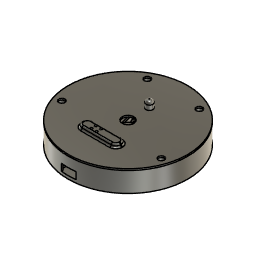
ViveTrackerPogoBatteryV2 (Autodesk Fusion 360 design; units mm, degrees)
Autodesk Fusion 360 part; units mm, degrees
sketch "CaseBase" plane through (0, 0, 0) normal (0, 0, 1) x (1, 0, 0)
  circle A0 centre (0, 0) radius 39
  dimension "d3" = 78
  constraint coincident A0.centre origin
  measures "d3" diameter of A0
sketch "Charging Module" plane through (0, 0, 0) normal (0, 0, 1) x (1, 0, 0)
  line L0 (-10, 37.25, 1) -> (10, 37.25, 1)
  line L1 (10, 37.25, 1) -> (10, 12.25, 1)
  line L2 (10, 12.25, 1) -> (-10, 12.25, 1)
  line L3 (-10, 12.25, 1) -> (-10, 37.25, 1)
  dimension "d9" = 25
  dimension "d10" = 20
sketch "Batteries" plane through (0, 0, 0) normal (0, 0, 1) x (1, 0, 0)
  line L0 (0, 2.5) -> (0, 20)
  line L1 (14.1047, 22.1855, 1) -> (1.1638, -26.1107, 1)
  line L2 (20.4823, -31.2871, 1) -> (33.4233, 17.0092, 1)
  line L3 (33.4233, 17.0092, 1) -> (14.1047, 22.1855, 1)
  line L4 (1.1638, -26.1107, 1) -> (20.4823, -31.2871, 1)
  line L5 (-1.1638, -26.1107, 1) -> (-20.4823, -31.2871, 1)
  line L6 (-20.4823, -31.2871, 1) -> (-33.4233, 17.0092, 1)
  line L7 (-14.1047, 22.1855, 1) -> (-1.1638, -26.1107, 1)
  line L8 (-33.4233, 17.0092, 1) -> (-14.1047, 22.1855, 1)
  dimension "d52" = 20
  dimension "d53" = 50
extrude "Extrude6" add sketch "Charging Module" along normal blind 2 contours L0 L1 L2 L3 in plane through (0, 0, 1) normal (0, 0, 1) makes body 1
sketch "Sketch11" plane through (0, 0, 3) normal (0, 0, 1) x (-1, 0, 0)
  line L0 (10, -12.25) -> (-10, -12.25)
  line L1 (-10, -12.25) -> (-10, -37.25)
  line L2 (-10, -37.25) -> (10, -37.25)
  line L3 (10, -37.25) -> (10, -12.25)
  line L4 (4.508, -37.25) -> (-4.492, -37.25)
  line L5 (-4.492, -37.25) -> (-4.492, -29.85)
  line L6 (-4.492, -29.85) -> (4.508, -29.85)
  line L7 (4.508, -29.85) -> (4.508, -37.25)
  dimension "d64" = 9
  dimension "d65" = 7.4
  constraint coincident L2 L4.start
  measures "d64" distance of L4.start L4.end
  measures "d65" distance of L4.start L6.end
extrude "Extrude12" add sketch "Sketch11" along normal blind 3 contours L2 L4 L5 L6 L7 bodies 1
extrude "Extrude7" add sketch "CaseBase" along normal blind 13 separate body makes body 2
shell "Shell2" thickness 1 removed faces 1 at (-7.0083, -19.4245, 13) on bodies 2
sketch "ScrewHoleThing" plane through (0, 0, 0) normal (0, 0, 1) x (1, 0, 0)
  circle A0 centre (0, 0) radius 6
  dimension "d28" = 12
  constraint coincident A0.centre origin
  measures "d28" diameter of A0
extrude "Extrude8" add sketch "ScrewHoleThing" along normal blind 8.5 bodies 2
hole "Hole5" at (0, 0, 8.5) direction (0, 0, -1) diameter 7.25 depth 10 tip angle 180 bodies 2
sketch "OG Comparison" plane through (0, 0, 0) normal (0, 0, 1) x (1, 0, 0)
  circle A0 centre (0, 0) radius 45
  dimension "d51" = 90
  constraint coincident A0.centre origin
  measures "d51" diameter of A0
extrude "Extrude9" add sketch "Batteries" along normal blind 10 separate body contours L1 L2 L3 L4 | L5 L6 L7 L8 in plane through (0, 0, 1) normal (0, 0, 1) makes body 3 at (16.2306, 4.3613, 1) makes body 4 at (-18.3565, -13.4629, 1)
sketch "SwitchCutout" plane through (0, 0, 0) normal (0, 1, 0) x (1, 0, 0)
  line L0 (-4.75, -6.5, -40.0305) -> (4.75, -6.5, -40.0305)
  line L1 (4.75, -6.5, -40.0305) -> (4.75, -2, -40.0305)
  line L2 (4.75, -2, -40.0305) -> (-4.75, -2, -40.0305)
  line L3 (-4.75, -2, -40.0305) -> (-4.75, -6.5, -40.0305)
  dimension "d56" = 9.5
  dimension "d57" = 4.5
extrude "Extrude10" cut sketch "SwitchCutout" along normal blind 4 contours L0 L1 L2 L3 in plane through (0, -40.0305, 0) normal (0, 1, 0) bodies 4 3 2
sketch "Sketch10" plane through (0, 0, 1) normal (0, 0, 1) x (-1, 0, 0)
  line L0 (-6, 38.15) -> (6, 38.15)
  line L1 (6, 38.15) -> (6, 32.15)
  line L2 (6, 32.15) -> (-6, 32.15)
  line L3 (-6, 32.15) -> (-6, 38.15)
  circle A0 centre (0, 0) radius 6
  circle A1 centre (0, 0) radius 38
  dimension "d60" = 12
  dimension "d61" = 6
  constraint horizontal L0
  constraint vertical L1
  constraint horizontal L2
  constraint vertical L3
  measures "d60" distance of L0.start L0.end
  measures "d61" distance of L0.start L2.end
extrude "Extrude11" add sketch "Sketch10" along normal blind 1 contours L1 L2 L3 A1 picked at (0.6692, 34.0823) bodies 2
sketch "Sketch12" plane through (0, 0, 1) normal (0, 0, 1) x (-1, 0, 0)
  line L0 (6, 37.5233) -> (6, 32.15)
  line L1 (6, 32.15) -> (-6, 32.15)
  line L2 (-6, 32.15) -> (-6, 37.5233)
  arc A0 (-6, 37.5233) -> (6, 37.5233) centre (0, 0) ccw
  line L3 (13.9813, -22.3263) -> (13.0154, -22.5851)
  line L4 (13.0154, -22.5851) -> (0.0745, 25.7112)
  line L5 (0.0745, 25.7112) -> (1.0404, 25.97)
  line L6 (1.0404, 25.97) -> (13.9813, -22.3263)
  line L7 (22.2661, 31.9239) -> (35.2071, -16.3724)
  line L8 (35.2071, -16.3724) -> (34.2411, -16.6313)
  line L9 (21.3002, 31.665) -> (22.2661, 31.9239)
  line L10 (34.2411, -16.6313) -> (21.3002, 31.665)
  circle A1 centre (0, 0) radius 6
  line L11 (20.3106, 32.0212) -> (0.9921, 26.8448)
  line L12 (0.9921, 26.8448) -> (0.7333, 27.8107)
  line L13 (0.7333, 27.8107) -> (20.0518, 32.9871)
  line L14 (20.0518, 32.9871) -> (20.3106, 32.0212)
  line L15 (0, -2.5) -> (0, -20)
  line L16 (-20.3106, 32.0212) -> (-0.9921, 26.8448)
  line L17 (-0.9921, 26.8448) -> (-0.7333, 27.8107)
  line L18 (-20.0518, 32.9871) -> (-20.3106, 32.0212)
  line L19 (-0.7333, 27.8107) -> (-20.0518, 32.9871)
  line L20 (-34.2411, -16.6313) -> (-21.3002, 31.665)
  line L21 (-21.3002, 31.665) -> (-22.2661, 31.9239)
  line L22 (-35.2071, -16.3724) -> (-34.2411, -16.6313)
  line L23 (-22.2661, 31.9239) -> (-35.2071, -16.3724)
  line L24 (-1.0404, 25.97) -> (-13.9813, -22.3263)
  line L25 (-13.9813, -22.3263) -> (-13.0154, -22.5851)
  line L26 (-0.0745, 25.7112) -> (-1.0404, 25.97)
  line L27 (-13.0154, -22.5851) -> (-0.0745, 25.7112)
  dimension "d68" = 50
  dimension "d69" = 1
  dimension "d70" = 50
  dimension "d71" = 1
  dimension "d86" = 20
  dimension "d87" = 1
  constraint symmetric L3.start L15 L24.end
  constraint symmetric L3.end L15 L25.end
  constraint symmetric L4.end L15 L26.start
  constraint symmetric L5.end L15 L24.start
  constraint symmetric L8.end L15 L20.start
  constraint symmetric L7.start L15 L21.end
  constraint symmetric L7.end L15 L22.start
  constraint symmetric L9.start L15 L20.end
  constraint symmetric L11.start L15 L16.start
  constraint symmetric L11.end L15 L16.end
  constraint symmetric L12.end L15 L17.end
  constraint symmetric L13.end L15 L18.start
  measures "d68" distance of L3.start L5.end
  measures "d69" distance of L3.start L3.end
  measures "d70" distance of L7.start L7.end
  measures "d71" distance of L8.end L7.end
  measures "d86" distance of L11.start L11.end
  measures "d87" distance of L11.end L12.end
extrude "Extrude16" add sketch "Sketch12" along normal blind 4 contours A0 L11 L12 L13 L14 | A0 L7 L10 | A0 L16 L17 L18 L19 | A0 L20 L23 | L3 L4 L5 L6 | L24 L25 L26 L27 bodies 2
sketch "Sketch14" plane through (0, 0, 1) normal (0, 0, 1) x (-1, 0, 0)
  line L0 (10.7, -36.7464) -> (10.2816, -36.7464)
  line L1 (10.2816, -36.7464) -> (10.2816, -12.3822)
  line L2 (10.2816, -12.3822) -> (10.7, -12.3822)
  line L3 (10.7, -12.3822) -> (10.7, -36.7464)
  line L4 (13.0154, -22.5851) -> (0.0745, 25.7112)
  line L5 (-10.3, -12.3822) -> (-10.3, -36.7464)
  line L6 (-10.3, -36.7464) -> (-10.7184, -36.7464)
  line L7 (-10.7184, -12.3822) -> (-10.3, -12.3822)
  line L8 (-10.7184, -36.7464) -> (-10.7184, -12.3822)
  circle A0 centre (8.7853, -10.6413) radius 1
  circle A1 centre (-8.7147, -10.6413) radius 1
  dimension "d78" = 2
  dimension "d79" = 2
  constraint horizontal L0
  constraint vertical L1
  constraint horizontal L2
  constraint vertical L3
  constraint coincident L1.end L4
  constraint horizontal L6
  constraint vertical L8
  constraint horizontal L7
  constraint vertical L5
  measures "d78" diameter of A0
  measures "d79" diameter of A1
sketch "Sketch15" plane through (0, 37.25, 0) normal (0, 1, 0) x (-1, 0, 0)
  line L0 (-10, 1) -> (10, 1)
  line L1 (10, 1) -> (10, 3)
  line L2 (10, 3) -> (4.508, 3)
  line L3 (4.508, 3) -> (4.508, 6)
  line L4 (4.508, 6) -> (-4.492, 6)
  line L5 (-4.492, 6) -> (-4.492, 3)
  line L6 (-4.492, 3) -> (-10, 3)
  line L7 (-10, 3) -> (-10, 1)
  line L8 (-7, 7.7333) -> (7, 7.7333)
  line L9 (7, 7.7333) -> (7, 1.7333)
  line L10 (7, 1.7333) -> (-7, 1.7333)
  line L11 (-7, 1.7333) -> (-7, 7.7333)
  line L12 (-7, 7.7333) -> (7, 1.7333) construction
  line L13 (7, 7.7333) -> (-7, 1.7333) construction
  point P0 (0, 4.7333)
  dimension "d80" = 14
  dimension "d81" = 6
  constraint horizontal L8
  constraint perpendicular L8 L9
  constraint parallel L8 L10
  constraint parallel L9 L11
  constraint coincident L12 P0
  constraint coincident L13 P0
  measures "d80" distance of L9.end L10.end
  measures "d81" distance of L8.end L9.end
extrude "Extrude14" cut sketch "Sketch15" along normal blind 3 contours L2 L3 L4 L5 L6 L8 L9 L11 | L2 L3 L4 L5 L6 L9 L10 L11 bodies 2 3 4
extrude "Extrude15" add sketch "Sketch14" along normal blind 1.5 contours L0 L1 L3 L4 | L4 A0 | L4 A0 | L5 L6 L7 L8 | A1 bodies 2 4 3
sketch "ScrewStands" plane through (0, 0, 1) normal (0, 0, 1) x (-1, 0, 0)
  line L0 (37.6453, 8.3508) -> (33.8865, 6.9827)
  line L1 (31.1503, 14.5003) -> (34.9091, 15.8684)
  line L2 (34.9091, 15.8684) -> (37.6453, 8.3508)
  line L3 (37.6453, 8.3508) -> (27.3916, 13.1322) construction
  line L4 (30.1277, 5.6146) -> (34.9091, 15.8684) construction
  arc A0 (28.7596, 9.3734) -> (33.8865, 6.9827) centre (32.5184, 10.7415) ccw
  arc A1 (31.1503, 14.5003) -> (28.7596, 9.3734) centre (32.5184, 10.7415) ccw
  arc A2 (14.9863, -26.1759) -> (13.5222, -31.64) centre (16.9863, -29.64) ccw
  arc A3 (20.4504, -27.64) -> (14.9863, -26.1759) centre (16.9863, -29.64) ccw
  line L5 (22.4504, -31.1041) -> (15.5222, -35.1041)
  line L6 (15.5222, -35.1041) -> (13.5222, -31.64)
  line L7 (20.4504, -27.64) -> (22.4504, -31.1041)
  line L8 (0, -2.5) -> (0, -20)
  line L9 (-15.5222, -35.1041) -> (-13.5222, -31.64)
  line L10 (-22.4504, -31.1041) -> (-15.5222, -35.1041)
  line L11 (-20.4504, -27.64) -> (-22.4504, -31.1041)
  arc A4 (-14.9863, -26.1759) -> (-20.4504, -27.64) centre (-16.9863, -29.64) ccw
  arc A5 (-13.5222, -31.64) -> (-14.9863, -26.1759) centre (-16.9863, -29.64) ccw
  arc A6 (-33.8865, 6.9827) -> (-28.7596, 9.3734) centre (-32.5184, 10.7415) ccw
  arc A7 (-28.7596, 9.3734) -> (-31.1503, 14.5003) centre (-32.5184, 10.7415) ccw
  line L12 (-34.9091, 15.8684) -> (-37.6453, 8.3508)
  line L13 (-37.6453, 8.3508) -> (-33.8865, 6.9827)
  line L14 (-31.1503, 14.5003) -> (-34.9091, 15.8684)
  point P0 (32.5184, 10.7415)
  dimension "d90" = 8
  dimension "d91" = 4
  dimension "d92" = 4
  dimension "d95" = 4
  dimension "d96" = 4
  constraint parallel L0 L1
  constraint coincident L3 P0
  constraint coincident L4 P0
  constraint coincident L4.start L0
  constraint tangent L0 A0
  constraint coincident L3.end L1
  constraint tangent L1 A1
  constraint coincident A0.start A1.end
  constraint parallel L6 L7
  constraint tangent A2 L6
  constraint tangent A3 L7
  constraint coincident A2.start A3.end
  constraint symmetric L0.start L8 L12.end
  constraint symmetric L1.end L8 L12.start
  constraint symmetric L0.end L8 A6.start
  constraint symmetric A0.start L8 A6.end
  constraint symmetric A0 L8 A6
  constraint symmetric L1.start L8 A7.end
  constraint symmetric A1 L8 A7
  constraint symmetric A2.start L8 A4.start
  constraint symmetric A2.end L8 L9.end
  constraint symmetric A3.start L8 L11.start
  constraint symmetric L5.start L8 L10.start
  constraint symmetric L5.end L8 L9.start
  constraint symmetric A2 L8 A5
  constraint symmetric A3 L8 A4
  measures "d90" distance of L3.end L1.end
  measures "d91" radius of A0
  measures "d92" radius of A1
  measures "d95" radius of A2
  measures "d96" radius of A3
extrude "Extrude17" add sketch "ScrewStands" along normal blind 12 bodies 2
sketch "Sketch17" plane through (0, 0, 13) normal (0, 0, 1) x (-1, 0, 0)
  line L0 (34.5826, 15.7495) -> (31.1503, 14.5003)
  arc A0 (31.1503, 14.5003) -> (33.8865, 6.9827) centre (32.5184, 10.7415) ccw
  line L1 (33.8865, 6.9827) -> (37.1141, 8.1575)
  line L2 (22.2695, -30.7907) -> (20.4504, -27.64)
  arc A1 (20.4504, -27.64) -> (13.5222, -31.64) centre (16.9863, -29.64) ccw
  line L3 (13.5222, -31.64) -> (15.3297, -34.7707)
  line L4 (-15.3297, -34.7707) -> (-13.5222, -31.64)
  arc A2 (-13.5222, -31.64) -> (-20.4504, -27.64) centre (-16.9863, -29.64) ccw
  line L5 (-20.4504, -27.64) -> (-22.2695, -30.7907)
  line L6 (-37.1141, 8.1575) -> (-33.8865, 6.9827)
  arc A3 (-33.8865, 6.9827) -> (-31.1503, 14.5003) centre (-32.5184, 10.7415) ccw
  line L7 (-31.1503, 14.5003) -> (-34.5826, 15.7495)
  circle A4 centre (16.9863, -29.64) radius 3
  circle A5 centre (32.5184, 10.7415) radius 3
  circle A6 centre (-16.9863, -29.64) radius 3
  circle A7 centre (-32.5184, 10.7415) radius 3
  circle A8 centre (0, 0) radius 39
  arc A9 (34.5826, 15.7495) -> (-34.5826, 15.7495) centre (0, 0) ccw
  arc A10 (22.2695, -30.7907) -> (37.1141, 8.1575) centre (0, 0) ccw
  arc A11 (-15.3297, -34.7707) -> (15.3297, -34.7707) centre (0, 0) ccw
  arc A12 (-37.1141, 8.1575) -> (-22.2695, -30.7907) centre (0, 0) ccw
  dimension "d97" = 6
  dimension "d98" = 6
  constraint concentric A1 A4
  constraint concentric A0 A5
  measures "d97" diameter of A4
  measures "d98" diameter of A5
hole "Hole6" at (-16.9863, 29.64, 13) at (-32.5184, -10.7415, 13) at (16.9863, 29.64, 13) at (32.5184, -10.7415, 13) direction (0, 0, -1) diameter 5.25 depth 8 tip angle 180 bodies 2
sketch "Sketch22" plane through (0, 0, 0) normal (0, 0, 1) x (1, 0, 0)
  circle A0 through (39, 0, 13) (-19.5, 33.775, 13) (-19.5, -33.775, 13)
  dimension "d109" = 78
extrude "Extrude18" add sketch "Sketch22" along normal blind 1 separate body contours A0 in plane through (0, 0, 13) normal (0, 0, 1) makes body 5
hole "Hole7" at (32.5184, -10.7415, 13) at (-32.5184, -10.7415, 13) at (-16.9863, 29.64, 13) at (16.9863, 29.64, 13) direction (0, 0, 1) diameter 4 depth 4 tip angle 180 bodies 5
hole "Hole8" at (0, 0, 0) direction (0, 0, 1) diameter 7.6 depth 20 tip angle 180 bodies 5
other "Base Mesh Feature2"
other "Modify5"
sketch "Sketch26" plane through (0, 0, 14) normal (0, 0, 1) x (-1, 0, 0)
  circle A0 centre (0, 0) radius 3.8
  circle A1 centre (16.9863, -29.64) radius 2
  circle A2 centre (-32.5184, 10.7415) radius 2
  circle A3 centre (32.5184, 10.7415) radius 2
  circle A4 centre (-16.9863, -29.64) radius 2
  circle A5 centre (0, 0) radius 39
  line L0 (-12.5, 20.5) -> (12.5, 20.5)
  line L1 (12.5, 20.5) -> (12.5, 14)
  line L2 (12.5, 14) -> (-12.5, 14)
  line L3 (-12.5, 14) -> (-12.5, 20.5)
  circle A6 centre (5.2594, 18.67) radius 0.75
  circle A7 centre (5.2594, 15.77) radius 0.75
  circle A8 centre (1.7594, 18.67) radius 0.75
  circle A9 centre (1.7594, 15.77) radius 0.75
  dimension "d126" = 1.5
  dimension "d127" = 1.5
  dimension "d128" = 1.5
  dimension "d129" = 1.5
  constraint horizontal L0
  constraint vertical L1
  constraint horizontal L2
  constraint vertical L3
  measures "d126" diameter of A6
  measures "d127" diameter of A7
  measures "d128" diameter of A8
  measures "d129" diameter of A9
sketch "Sketch27" plane through (0, 0, 14) normal (0, 0, 1) x (-1, 0, 0)
  circle A0 centre (0, -14) radius 2.25
  dimension "d124" = 4.5
  measures "d124" diameter of A0
extrude "Extrude20" add sketch "Sketch27" along normal blind 5 bodies 5
fillet "Fillet1" radius 2 1 edges at (2.0977, 14.8136, 19) on bodies 5
extrude "Extrude21" add sketch "Sketch26" along normal blind 2 contours L0 L1 L2 L3 | A6 | A7 | A8 | A9 bodies 5
fillet "Fillet2" radius 3 4 edges at (12.5, -14, 15) (12.5, -20.5, 15) (-12.5, -14, 15) (-12.5, -20.5, 15) on bodies 5
fillet "Fillet3" radius 1 8 faces at (12.5, -17.1667, 14.6667) (9.7852, -14.0136, 15.3333) (-3.1667, -14, 15.3333) (-9.7852, -14.0136, 15.3333) (-12.5, -17.3333, 14.6667) (-11.3545, -19.8582, 14.6667) (3.1667, -20.5, 15.3333) (11.3545, -19.8582, 14.6667) on bodies 5
hole "Hole9" at (-1.7594, -18.67, 14) at (-1.7594, -15.77, 14) at (-5.2594, -15.77, 14) at (-5.2594, -18.67, 14) direction (0, 0, -1) diameter 1.5 depth 3.2 tip angle 180 bodies 5
extrude "Extrude22" cut sketch "Sketch26" along normal blind 2.5 and the other way blind 1.55 contours A6 | A7 | A8 | A9 bodies 5
combine "Combine1" operation cut target body 2 tool bodies 1 keep tools
hidden bodies 1 3 4
named bodies: "Charging Module", "LowerCase", "Batt1", "Batt2", "TopLidBase"
